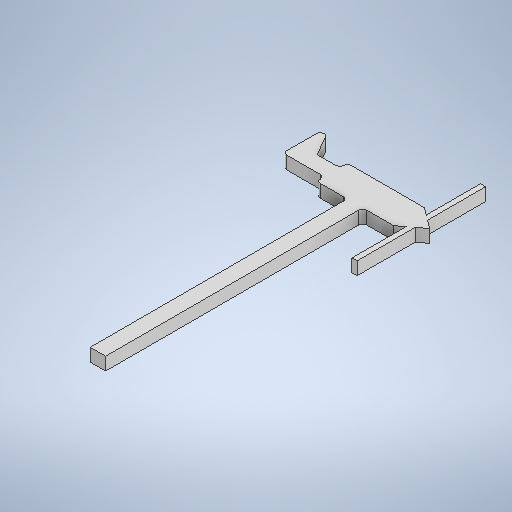
# Autodesk Inventor part: Nacrt
Saved by Autodesk Inventor 2025.2 (Build 292293000, 293)
## iProperties
Created: 2025-12-19
Part Number: Nacrt
Material: Všeobecné
Document SubType Name: Modeling
Designer: kozna
Density: 1 g/cm^3
Appearance: Výchozí
Author: kozna
Autodesk Inventor part; units mm, degrees
ref_plane "YZ Plane" through (0, 0, 0) normal (1, 0, 0) x (0, 1, 0)
ref_plane "XZ Plane" through (0, 0, 0) normal (0, 1, 0) x (-1, 0, 0)
ref_plane "XY Plane" through (0, 0, 0) normal (0, 0, 1) x (1, 0, 0)
sketch "Náčrt1" plane through (0, 0, 0) normal (0, 1, 0) x (-1, 0, 0)
  line L0 (30, -485) -> (30, 500)
  line L1 (30, 500) -> (-30, 500)
  line L2 (-30, 500) -> (-30, -485)
  line L3 (-338.3956, 0) -> (421.6903, 0) projected
  line L4 (0, -1072.3) -> (0, 762.05) projected
  line L5 (45, -500) -> (135, -500)
  line L6 (150, -605.5) -> (150, -605.5)
  line L7 (135, -620.5) -> (-150, -620.5)
  line L8 (-150, -620.5) -> (-150, -500)
  line L9 (-178, -810.25) -> (-198, -810.25)
  line L10 (-198, -810.25) -> (-198, -310.25)
  line L11 (-198, -310.25) -> (-178, -310.25)
  line L12 (-178, -310.25) -> (-178, -810.25)
  line L13 (-150, -620.5) -> (-229.8119, -560.25)
  line L14 (-229.8119, -560.25) -> (-150, -500)
  line L15 (165, -590.5) -> (310, -590.5)
  line L16 (310, -590.5) -> (310, -545)
  line L17 (295, -530) -> (165, -530)
  line L18 (310, -590.5) -> (310, -660.0929)
  line L19 (282.0096, -667.5929) -> (237.5, -590.5)
  arc A0 (135, -620.5) -> (150, -605.5) centre (135, -605.5) ccw
  arc A1 (165, -590.5) -> (150, -605.5) centre (165, -605.5) ccw
  line L20 (150, -515) -> (150, -515)
  arc A2 (150, -515) -> (135, -500) centre (135, -515) ccw
  arc A3 (150, -515) -> (165, -530) centre (165, -515) ccw
  arc A4 (310, -545) -> (295, -530) centre (295, -545) ccw
  arc A5 (30, -485) -> (45, -500) centre (45, -485) ccw
  line L21 (-45, -500) -> (-150, -500)
  arc A6 (-45, -500) -> (-30, -485) centre (-45, -485) ccw
  line L22 (45, -500) -> (-45, -500)
  arc A7 (282.0096, -667.5929) -> (310, -660.0929) centre (295, -660.0929) ccw
  point P0 (0, 0)
  point P1 (150, -620.5)
  point P2 (150, -500)
  point P3 (310, -530)
  point P4 (150, -530)
  point P5 (-178, -521.1372)
  point P6 (-198, -536.2352)
  point P7 (-198, -584.2648)
  point P8 (-178, -599.3628)
  dimension "d0" = 60
  dimension "d2" = 300
  dimension "d3" = 120.5
  dimension "d4" = 20
  dimension "d5" = 500
  dimension "d7" = 189.75
  dimension "d9" = 100
  dimension "d11" = 100
  dimension "d12" = 178
  dimension "d13" = 160
  dimension "d14" = 30
  dimension "d15" = 30
  dimension "d16" = 30
  dimension "d17" = 15
  dimension "d18" = 15
  dimension "d19" = 15
  dimension "d20" = 15
  dimension "d21" = 15
  dimension "d22" = 1000
  dimension "d23" = 15
  constraints: 42 end point, 17 tangent, 16 point on circle, 11 point on line, 8 centre point, 6 parallel, 5 horizontal, 3 perpendicular, 2 equal radius, 2 vertical, 1 midpoint, 3 other
  measures "d0" distance of L0.end L1.end
  measures "d2" distance of point (150, -620.5) L7.end
  measures "d3" distance of point (150, -500) point (150, -620.5)
  measures "d4" distance of L10.end L11.end
  measures "d5" distance of L9.end L10.end
  measures "d7" distance between parallel lines of L7 L9
  measures "d9" distance of L7.end L13.end
  measures "d11" distance of L13.end L8.end
  measures "d12" distance between parallel lines of L12 L4
  measures "d13" distance of point (310, -530) point (150, -530)
  measures "d14" distance between parallel lines of L7 L15
  measures "d15" distance between parallel lines of L5 L17
  measures "d16" angle of L19 L18
  measures "d17" radius of A0
  measures "d18" radius of A2
  measures "d19" radius of A4
  measures "d20" radius of A5
  measures "d21" radius of A6
  measures "d22" distance between parallel lines of L1 L22
  measures "d23" radius of A7
extrude "Vysunutí1" add sketch "Náčrt1" along normal blind 50
